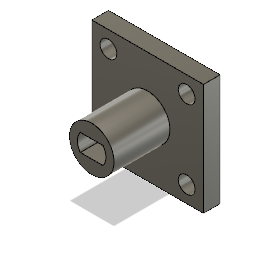
Roue 2D (Autodesk Fusion 360 archive; units mm, degrees)
design "Fixation"
Autodesk Fusion 360 part; units mm, degrees
sketch "Sketch1" plane through (0, 0, 0) normal (0, 0, 1) x (1, 0, 0)
  line L0 (2.55, 1.55) -> (-2.55, -1.55) construction
  line L1 (2.55, 1.55) -> (-2.55, -1.55) construction
  line L2 (-2.55, 1.55) -> (-2.55, -1.55)
  circle A0 centre (0, 0) radius 4
  line L3 (-2.55, 1.55) -> (2.55, -1.55) construction
  line L4 (-2.55, -1.55) -> (2.55, -1.55)
  line L5 (2.55, 1.55) -> (-2.55, 1.55)
  line L6 (2.55, 1.55) -> (-2.55, -1.55) construction
  line L7 (-2.55, 1.55) -> (2.55, -1.55) construction
  line L8 (-2.55, 1.55) -> (2.55, -1.55) construction
  circle A1 centre (0, 0) radius 2.55
  line L9 (2.55, -1.55) -> (2.55, 1.55)
  line L10 (-10, 10) -> (10, 10)
  line L11 (10, 10) -> (10, -10)
  line L12 (10, -10) -> (-10, -10)
  line L13 (-10, -10) -> (-10, 10)
  circle A2 centre (-7, 7) radius 1.5
  line L14 (0, 10) -> (0, 7.5)
  circle A3 centre (7, 7) radius 1.5
  line L15 (-10, 0) -> (-8.5, 0)
  circle A4 centre (-7, -7) radius 1.5
  circle A5 centre (7, -7) radius 1.5
  dimension "d1" = 5.1
  dimension "d2" = 5.1
  dimension "d3" = 3.1
  dimension "d4" = 8
  dimension "d5" = 5.1
  dimension "d6" = 5.1
  dimension "d7" = 20
  dimension "d8" = 20
  dimension "d9" = 3
  measures "d4" diameter of A0
  measures "d5" diameter of A1
  measures "d9" diameter of A2
extrude "Extrude1" add sketch "Sketch1" along normal blind 10 contours L2 L5 A1 | L2 L4 A1 | L5 A1 | L4 A1 | L5 A1 L9 | L4 A1 L9 | A0 makes body 1
extrude "Extrude2" add sketch "Sketch1" against normal blind 3 separate body contours L10 L11 L12 L13 makes body 2
extrude "Extrude3" add sketch "Sketch1" against normal blind 3 contours L2 L5 A1 | L2 L4 A1 | L4 L5 A1 | L5 A1 | L4 A1 | L5 A1 L9 | L4 A1 L9 | A0 bodies 1 2
